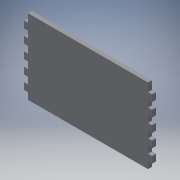
# Autodesk Inventor part: полуверх
Saved by Autodesk Inventor 2019 (Build 230136000, 136)
## iProperties
Created: 2022-02-24
Part Number: полуверх
Material: Типовые
Document SubType Name: Modeling
Designer: korsh
Density: 1 g/cm^3
Appearance: По умолчанию
Author: korsh
Autodesk Inventor part; units mm, degrees
ref_plane "YZ Plane" through (0, 0, 0) normal (1, 0, 0) x (0, 1, 0)
ref_plane "XZ Plane" through (0, 0, 0) normal (0, 1, 0) x (-1, 0, 0)
ref_plane "XY Plane" through (0, 0, 0) normal (0, 0, 1) x (1, 0, 0)
sketch "Эскиз1" plane through (0, 0, 0) normal (0, 0, 1) x (1, 0, 0)
  line L0 (0, 0) -> (0, 10) projected
  line L1 (0, 0) -> (6, 0) projected
  line L2 (6, 10) -> (6, 0) projected
  line L3 (0, 10) -> (6, 10) projected
  line L4 (0, -20) -> (0, -10) projected
  line L5 (0, -20) -> (6, -20) projected
  line L6 (6, -10) -> (6, -20) projected
  line L7 (0, -10) -> (6, -10) projected
  line L8 (0, -40) -> (0, -30) projected
  line L9 (0, -40) -> (6, -40) projected
  line L10 (6, -30) -> (6, -40) projected
  line L11 (0, -30) -> (6, -30) projected
  line L12 (0, -60) -> (0, -50) projected
  line L13 (0, -60) -> (6, -60) projected
  line L14 (6, -50) -> (6, -60) projected
  line L15 (0, -50) -> (6, -50) projected
  line L16 (0, -80) -> (0, -70) projected
  line L17 (0, -80) -> (6, -80) projected
  line L18 (6, -70) -> (6, -80) projected
  line L19 (0, -70) -> (6, -70) projected
  line L20 (6, 22.5234) -> (6, 9.9924) projected
  line L21 (6, -80) -> (6, -90) projected
  line L22 (186, 9.9924) -> (186, 22.5234) projected
  line L23 (186, 0) -> (186, 10) projected
  line L24 (186, 0) -> (192, 0) projected
  line L25 (192, 10) -> (192, 0) projected
  line L26 (186, 10) -> (192, 10) projected
  line L27 (186, -20) -> (186, -10) projected
  line L28 (186, -20) -> (192, -20) projected
  line L29 (192, -10) -> (192, -20) projected
  line L30 (186, -10) -> (192, -10) projected
  line L31 (186, -40) -> (186, -30) projected
  line L32 (186, -40) -> (192, -40) projected
  line L33 (192, -30) -> (192, -40) projected
  line L34 (186, -30) -> (192, -30) projected
  line L35 (186, -60) -> (186, -50) projected
  line L36 (186, -60) -> (192, -60) projected
  line L37 (192, -50) -> (192, -60) projected
  line L38 (186, -50) -> (192, -50) projected
  line L39 (186, -80) -> (186, -70) projected
  line L40 (186, -80) -> (192, -80) projected
  line L41 (192, -70) -> (192, -80) projected
  line L42 (186, -70) -> (192, -70) projected
  line L43 (186, -90) -> (186, -80) projected
  line L44 (186, 22.5234) -> (6, 22.5234)
  line L45 (6, 22.5234) -> (6, -90)
  line L46 (6, -90) -> (186, -90)
  line L47 (186, -90) -> (186, 22.5234)
  constraints: 8 end point, 2 parallel, 1 horizontal, 1 perpendicular
extrude "Выдавливание1" add sketch "Эскиз1" along normal blind 6
